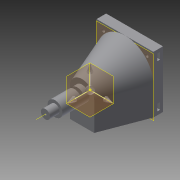
# Autodesk Inventor part: Power_Meter_Adapter_Part1
Saved by Autodesk Inventor 2015 (Build 190159000, 159)
## iProperties
Created: 2015-02-18
Part Number: Power_Meter_Adapter_Part1
Material: Generic
Document SubType Name: Modeling
Designer: sgneitin
Density: 1 g/cm^3
Appearance: Default
Author: sgneitin
Autodesk Inventor part; units mm, degrees
ref_plane "YZ Plane" through (0, 0, 0) normal (1, 0, 0) x (0, 1, 0)
ref_plane "XZ Plane" through (0, 0, 0) normal (0, 1, 0) x (-1, 0, 0)
sketch "Sketch2" plane through (0, 0, 0) normal (0, 0, 1) x (1, 0, 0)
  line L0 (-29.75, 59.5) -> (29.75, 59.5)
  line L1 (29.75, 59.5) -> (29.75, 0)
  line L2 (29.75, 0) -> (-29.75, 0)
  line L3 (-29.75, 0) -> (-29.75, 59.5)
  point P0 (0, 0)
  point P1 (0, 0)
  dimension "d0" = 59.5
  constraints: 8 end point, 2 parallel, 2 perpendicular, 1 coincident, 1 horizontal, 1 midpoint
  measures "d0" distance of L2.end L0.start
extrude "Extrusion1" add sketch "Sketch2" along normal blind 55
sketch "Sketch3" plane through (0, 0, 55) normal (0, 0, 1) x (1, 0, 0)
  circle A0 centre (0, 29.75) radius 1
  circle A1 centre (0, 29.75) radius 7.75
  line L0 (0, 0) -> (0, 59.5) construction
  line L1 (29.75, 59.5) -> (-29.75, 59.5) construction
  line L2 (29.75, 0) -> (29.75, 59.5) construction
  line L3 (29.75, 29.75) -> (-29.75, 29.75) construction
  line L4 (-29.75, 59.5) -> (-29.75, 0) construction
  line L5 (-29.75, 0) -> (29.75, 0) projected
  dimension "d3" = 15.5
  dimension "d5" = 2
  dimension "d47" = 22
  constraints: 5 midpoint, 4 end point, 2 centre point, 1 concentric
  measures "d3" diameter of A1
  measures "d5" diameter of A0
  measures "d47" distance edge to line of A1 L5
extrude "Extrusion2" add sketch "Sketch3" along normal blind 28.3
sketch "Sketch4" plane through (0, 29.75, 83.3) normal (0, 0, 1) x (1, 0, 0)
  circle A0 centre (0, 0) radius 1
  circle A1 centre (0, 0) radius 4.75
  circle A2 centre (0, 0) radius 1 projected
  point P0 (0, -29.75)
  dimension "d8" = 9.5
  constraints: 3 concentric, 2 centre point
  measures "d8" diameter of A1
extrude "Extrusion3" add sketch "Sketch4" along normal blind 10
sketch "Sketch10" plane through (0, 0, 0) normal (0, 0, -1) x (-1, 0, 0)
  circle A0 centre (-22.75, 52.5) radius 1.75
  circle A1 centre (-22.75, 7) radius 1.75
  circle A2 centre (22.75, 52.5) radius 1.75
  circle A3 centre (22.75, 7) radius 1.75
  line L0 (-29.75, 59.5) -> (-29.75, 0) projected
  line L1 (29.75, 59.5) -> (-29.75, 59.5) projected
  line L2 (-29.75, 29.75) -> (29.75, 29.75) construction
  line L3 (29.75, 0) -> (29.75, 59.5) construction
  line L4 (0, 59.5) -> (0, 0) construction
  dimension "d29" = 7
  dimension "d30" = 7
  dimension "d33" = 3.5
  constraints: 4 centre point, 4 end point, 3 equal radius, 3 midpoint, 2 symmetric about line, 1 vertical, 1 other
  measures "d29" distance from line of L0 A0.centre
  measures "d30" distance from line of A0.centre L1
  measures "d33" diameter of A0
extrude "Extrusion5" cut sketch "Sketch10" against normal blind 10
sketch "Sketch9" plane through (29.75, 0, 0) normal (1, 0, 0) x (0, 0, -1)
  line L0 (-6, 56) -> (-3, 56)
  line L1 (-3, 56) -> (-3, 49)
  line L2 (-3, 49) -> (-6, 49)
  line L3 (-6, 49) -> (-6, 56)
  line L4 (-6, 10.5) -> (-3, 10.5)
  line L5 (-3, 10.5) -> (-3, 3.5)
  line L6 (-3, 3.5) -> (-6, 3.5)
  line L7 (-6, 3.5) -> (-6, 10.5)
  line L8 (0, 59.5) -> (-55, 59.5) projected
  line L9 (-55, 0) -> (-55, 59.5) construction
  line L10 (-55, 29.75) -> (0, 29.75) construction
  line L11 (0, 0) -> (0, 59.5) construction
  line L12 (0, 54.25) -> (0, 50.75) projected
  line L13 (0, 52.5) -> (-10, 52.5) construction
  line L14 (-10, 54.25) -> (-10, 50.75) projected
  dimension "d24" = 7
  dimension "d25" = 3
  dimension "d26" = 3
  constraints: 20 end point, 4 midpoint, 4 parallel, 2 equal length, 2 horizontal, 2 perpendicular, 1 point on line, 2 other
  measures "d24" distance of L2.end L0.start
  measures "d25" distance of L1.end L2.end
  measures "d26" distance between parallel lines of L11 L1
extrude "Extrusion4" cut sketch "Sketch9" against normal blind 10
mirror "Mirror1" about plane through (0, 0, 0) normal (1, 0, 0) of "Extrusion4"
ref_plane "Work Plane1" through (0, 0, 10) normal (0, 0, 1) x (1, 0, 0)
sketch "Sketch11" plane through (0, 0, 10) normal (0, 0, 1) x (1, 0, 0)
  circle A0 centre (0, 29.75) radius 24.75
  circle A1 centre (0, 29.75) radius 1 projected
  line L0 (-29.75, 59.5) -> (29.75, 59.5) projected
  point P0 (0, 0)
  dimension "d49" = 5
  constraints: 1 centre point, 1 concentric
  measures "d49" distance edge to line of A0 L0
extrude "Extrusion6" cut sketch "Sketch11" against normal through all contours A0 | A1
loft "Loft2" cut section 1 edges at (-24.75, 29.75, 10) section 2 edges at (-1, 29.75, 55)
sketch "Sketch7" plane through (-29.75, 59.5, 0) normal (0, 1, 0) x (1, 0, 0)
  line L0 (35.75, -60) -> (23.75, -60)
  line L1 (23.75, -60) -> (23.75, -63)
  line L2 (23.75, -63) -> (35.75, -63)
  line L3 (35.75, -63) -> (35.75, -60)
  line L4 (29.75, -60) -> (29.75, -63) construction
  line L5 (26.5, -55) -> (28.5, -55) construction
  line L6 (29.75, -55) -> (29.75, -83.3) construction
  line L7 (59.5, -55) -> (0, -55) construction
  line L8 (22, -83.3) -> (37.5, -83.3) projected
  point P0 (29.75, 0)
  dimension "d16" = 3
  dimension "d17" = 12
  dimension "d18" = 5
  constraints: 12 end point, 4 midpoint, 2 parallel, 1 coincident, 1 collinear, 1 horizontal, 1 perpendicular
  measures "d16" distance of L2.end L0.start
  measures "d17" distance of L1.end L2.end
  measures "d18" distance between parallel lines of L7 L0
extrude "Extrusion7" cut sketch "Sketch7" against normal blind 32
sketch "Sketch12" plane through (-29.75, 27.5, 0) normal (0, 1, 0) x (1, 0, 0)
  line L0 (32.75, -60) -> (26.75, -60)
  line L1 (26.75, -60) -> (26.75, -63)
  line L2 (26.75, -63) -> (32.75, -63)
  line L3 (32.75, -63) -> (32.75, -60)
  line L4 (35.75, -60) -> (35.75, -63) projected
  line L5 (35.75, -63) -> (23.75, -63) projected
  line L6 (28.75, -60) -> (30.75, -60) construction
  line L7 (29.75, -60) -> (29.75, -63) construction
  line L8 (30.75, -63) -> (28.75, -63) construction
  point P0 (29.75, 0)
  point P1 (22.3338, -63)
  dimension "d44" = 6
  constraints: 10 end point, 3 parallel, 2 midpoint, 1 collinear, 1 horizontal, 1 perpendicular, 1 other
  measures "d44" distance between parallel lines of L1 L3
extrude "Extrusion8" cut sketch "Sketch12" against normal through all
sketch "Sketch14" plane through (0, 0, 0) normal (1, 0, 0) x (0, 1, 0)
  line L0 (59.5, 10) -> (42.5, 55)
  line L1 (42.5, 55) -> (79.5, 55)
  line L2 (79.5, 10) -> (79.5, 55)
  line L3 (59.5, 55) -> (0, 55) projected
  line L4 (37.5, 55) -> (37.5, 83.3) projected
  line L5 (59.5, 0) -> (59.5, 55) projected
  line L6 (5, 10) -> (54.5, 10) projected
  line L7 (79.5, 10) -> (59.5, 10)
  line L8 (59.5, 0) -> (59.5, 55) projected
  line L9 (54.25, 10) -> (50.75, 10) projected
  line L10 (29.75, -18.66) -> (29.75, 111.96) projected
  point P0 (0, 0)
  point P1 (55, 37.5)
  point P2 (55, 37.5)
  dimension "d54" = 5
  dimension "d55" = 20
  constraints: 8 end point, 5 point on line, 2 perpendicular, 1 collinear
  measures "d54" distance of L4.start L0.end
  measures "d55" distance of L2.start L0.start
revolve "Revolution1" cut sketch "Sketch14" angle 180 mid plane about axis through (0, 29.75, 55) along (0, 0, 1)
sketch "Sketch15" plane through (12.75, 29.75, 55) normal (0, 1, 0) x (1, 0, 0)
  line L0 (-42.5, 0) -> (-25.5, 0)
  line L1 (-25.5, 0) -> (0, 0)
  line L2 (-42.5, 0) -> (17, 0) projected
  line L3 (0, 0) -> (17, 0)
  line L4 (17, 0) -> (17, 45)
  line L5 (17, 55) -> (17, 0) projected
  line L6 (0, 0) -> (17, 45)
  line L7 (0, 0) -> (17, 45) projected
  line L8 (17, 45) -> (-25.5, 0)
  line L9 (-25.5, 0) -> (-42.5, 45)
  line L10 (-42.5, 45) -> (-25.5, 0) projected
  line L11 (-42.5, 0) -> (-42.5, 45)
  line L12 (-42.5, 55) -> (-42.5, 0) projected
  point P0 (-12.75, 55)
  constraints: 16 end point, 5 collinear, 1 horizontal
extrude "Extrusion10" cut sketch "Sketch15" against normal through all contours L11 L9 L0 | L6 L4 L2
body "Solid1"
